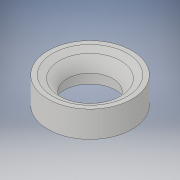
# Autodesk Inventor part: Graphite
Saved by Autodesk Inventor 2017 (Build 210142000, 142)
## iProperties
Created: 2016-07-19
Part Number: Graphite
Material: Generic
Document SubType Name: Modeling
Designer: Bill
Density: 1 g/cm^3
Appearance: Default
Author: Bill
Autodesk Inventor part; units mm, degrees
ref_plane "YZ Plane" through (0, 0, 0) normal (1, 0, 0) x (0, 1, 0)
ref_plane "XZ Plane" through (0, 0, 0) normal (0, 1, 0) x (-1, 0, 0)
ref_plane "XY Plane" through (0, 0, 0) normal (0, 0, 1) x (1, 0, 0)
sketch "Sketch1" plane through (0, 0, 0) normal (0, 0, 1) x (1, 0, 0)
  line L0 (-52.8574, -21.6553) -> (-32.6136, -21.6553)
  line L1 (-32.6136, -21.6553) -> (-28.702, -7.057)
  line L2 (-52.8574, -21.6553) -> (-52.8574, 11.3647)
  line L3 (-52.8574, 11.3647) -> (-47.8536, 11.3647) construction
  line L4 (0, -28.2593) -> (0, 17.9687) projected
  line L5 (-52.8574, 11.3647) -> (-46.9749, 11.3647)
  line L6 (-46.9749, 11.3647) -> (-38.6785, 7.496)
  arc A0 (-28.702, -7.057) -> (-38.6785, 7.496) centre (-51.804, -12.198) ccw
  point P0 (0, 0)
  dimension "d0" = 105
  dimension "d1" = 20.2438
  dimension "d2" = 32.6136
  dimension "d3" = 28.702
  dimension "d4" = 33.02
  dimension "d9" = 5.0038
  dimension "d10" = 25
  constraints: 12 end point, 2 horizontal, 2 point on circle, 1 centre point, 1 point on line, 1 vertical
  measures "d0" angle of L0 L1
  measures "d1" distance of L0.start L0.end
  measures "d2" horizontal distance of point (0, 0) L0.end
  measures "d3" horizontal distance of point (0, 0) L1.end
  measures "d4" distance of L0.start L2.end
  measures "d9" distance of L2.end L3.end
  measures "d10" angle of L3 L6
revolve "Revolution1" add sketch "Sketch1" angle 360 about axis through (0, -10, 0) along (0, 1, 0)
body "Solid1"
